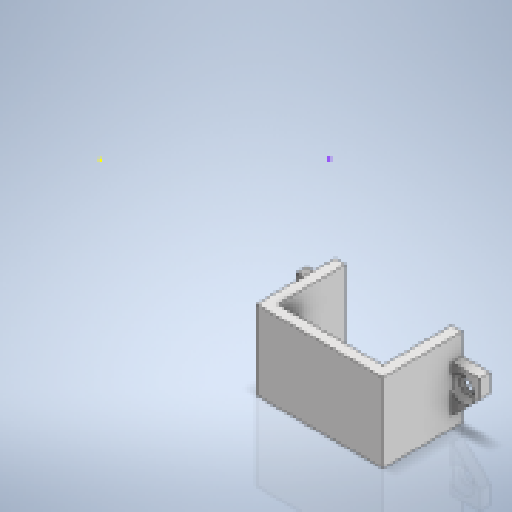
# Autodesk Inventor part: protetor_luz
Saved by Autodesk Inventor 2024.3 (Build 283343000, 343)
## iProperties
Created: 2024-05-17
Part Number: protetor_luz
Material: Genérico
Document SubType Name: Modeling
Designer: joaov
Density: 1 g/cm^3
Appearance: Padrão
Author: joaov
Autodesk Inventor part; units mm, degrees
ref_plane "YZ Plane" through (0, 0, 0) normal (1, 0, 0) x (0, 1, 0)
ref_plane "XZ Plane" through (0, 0, 0) normal (0, 1, 0) x (-1, 0, 0)
ref_plane "XY Plane" through (0, 0, 0) normal (0, 0, 1) x (1, 0, 0)
sketch "Esboço4" plane through (0, 0, 0) normal (0, 0, 1) x (1, 0, 0)
  point P0 (0, 0)
  point P1 (43.221, 21.8373)
  point P2 (101.0161, 22.7479)
  point P3 (77.0161, 22.7479)
sketch "Esboço5" plane through (0, 0, 0) normal (0, 0, 1) x (1, 0, 0)
  line L0 (46.357, -8.7268) -> (46.357, 6.1732)
  line L1 (66.357, 6.1732) -> (66.357, -8.7268)
  line L2 (46.357, 6.1732) -> (44.357, 6.1732)
  line L3 (44.357, 6.1732) -> (44.357, -8.7268)
  line L4 (44.357, -8.7268) -> (46.357, -8.7268)
  line L5 (56.357, 6.1732) -> (56.357, -8.7268)
  circle A0 centre (42.407, -1.2768) radius 1.4
  line L6 (39.007, -1.2768) -> (44.357, -6.6268)
  line L7 (39.007, -1.2768) -> (46.573, -1.2768) construction
  line L8 (39.007, -1.2768) -> (39.007, 2.1232)
  line L9 (39.007, 2.1232) -> (44.357, 2.1232)
  line L10 (66.357, -8.7268) -> (66.357, 6.1732)
  line L11 (66.357, 6.1732) -> (68.357, 6.1732)
  line L12 (68.357, 6.1732) -> (68.357, -8.7268)
  line L13 (68.357, -8.7268) -> (66.357, -8.7268)
  circle A1 centre (70.307, -1.2768) radius 1.4
  line L14 (73.707, -1.2768) -> (68.357, -6.6268)
  line L15 (73.707, -1.2768) -> (66.1409, -1.2768) construction
  line L16 (73.707, -1.2768) -> (73.707, 2.1232)
  line L17 (73.707, 2.1232) -> (68.357, 2.1232)
  point P0 (0, 0)
  dimension "d23" = 20
  dimension "d29" = 2
  dimension "d35" = 45
  constraints: 36 end point, 8 symmetric about line, 4 point on line, 3 perpendicular, 2 centre point, 2 horizontal, 1 equal length, 1 vertical, 1 other
  measures "d23" distance of L1.end L0.start
  measures "d29" distance of L0.end L2.end
  measures "d35" angle of L6 L7
extrude "Extrusão4" add sketch "Esboço5" along normal blind 2
sketch "Esboço6" plane through (0, 0, 2) normal (0, 0, 1) x (1, 0, 0)
  line L0 (46.357, 6.1732) -> (44.357, 6.1732) projected
  line L1 (46.357, 6.1732) -> (44.357, 6.1732)
  line L2 (44.357, -8.7268) -> (46.357, -8.7268) projected
  line L3 (46.357, -8.7268) -> (46.357, 6.1732)
  line L4 (44.357, 6.1732) -> (44.357, -8.7268)
  line L5 (46.357, -8.7268) -> (44.357, -8.7268)
  line L6 (66.357, 6.1732) -> (66.357, -8.7268) projected
  line L7 (68.357, 6.1732) -> (66.357, 6.1732) projected
  line L8 (66.357, 6.1732) -> (68.357, 6.1732)
  line L9 (68.357, 6.1732) -> (68.357, -8.7268)
  line L10 (68.357, -8.7268) -> (66.357, -8.7268)
  line L11 (66.357, -8.7268) -> (66.357, 6.1732)
  point P0 (0, 0)
  constraints: 16 end point, 4 perpendicular, 3 collinear, 1 vertical
extrude "Extrusão5" add sketch "Esboço6" along normal blind 11
sketch "Esboço7" plane through (0, 0, 13) normal (0, 0, 1) x (1, 0, 0)
  line L0 (44.357, 6.1732) -> (44.357, 2.1232) projected
  line L1 (68.357, -8.7268) -> (68.357, 6.1732) projected
  line L2 (44.357, 6.1732) -> (68.357, 6.1732)
  line L3 (68.357, 6.1732) -> (68.357, -8.7268)
  line L4 (68.357, -8.7268) -> (44.357, -8.7268)
  line L5 (44.357, -8.7268) -> (44.357, 6.1732)
  point P0 (0, 0)
  constraints: 8 end point, 2 parallel, 1 horizontal, 1 perpendicular
extrude "Extrusão6" add sketch "Esboço7" along normal blind 2
chamfer "Chanfro1" distance 1 angle 45 1 edges at (68.907, -1.2768, 2)
chamfer "Chanfro2" distance 1 angle 45 1 edges at (41.007, -1.2768, 2)
